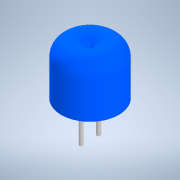
# Autodesk Inventor part: LED
Saved by Autodesk Inventor 2021 (Build 250183000, 183)
## iProperties
Created: 2021-06-29
Part Number: LED
Material: Generic
Document SubType Name: Modeling
Designer: shifa
Density: 1 g/cm^3
Appearance: Default
Author: shifa
Autodesk Inventor part; units mm, degrees
ref_plane "YZ Plane" through (0, 0, 0) normal (1, 0, 0) x (0, 1, 0)
ref_plane "XZ Plane" through (0, 0, 0) normal (0, 1, 0) x (-1, 0, 0)
ref_plane "XY Plane" through (0, 0, 0) normal (0, 0, 1) x (1, 0, 0)
sketch "Sketch1" plane through (0, 0, 0) normal (0, 0, 1) x (1, 0, 0)
  line L0 (3, -6.7347) -> (-5, -6.7347)
  line L1 (-5, -6.7347) -> (-5, 3.2653)
  line L2 (-1, 7.2653) -> (-1, 7.2653)
  line L3 (3, 3.2653) -> (3, -6.7347)
  arc A0 (3, 3.2653) -> (-1, 7.2653) centre (-1, 3.2653) ccw
  arc A1 (-1, 7.2653) -> (-5, 3.2653) centre (-1, 3.2653) ccw
  point P0 (0, 0)
  point P1 (-5, 7.2653)
  point P2 (3, 7.2653)
  point P3 (-1, 7.2653)
  dimension "d0" = 8
  dimension "d1" = 14
  dimension "d2" = 4
  constraints: 8 end point, 4 point on circle, 4 point on line, 4 tangent, 2 centre point, 2 parallel, 1 concentric, 1 horizontal, 1 perpendicular
  measures "d0" distance of point (-5, 7.265) point (3, 7.265)
  measures "d1" distance of L0.end point (-5, 7.265)
  measures "d2" radius of A0
revolve "Revolution1" add sketch "Sketch1" angle 360 about axis through (3, 3.2653, 0) along (0, -1, 0)
sketch "Sketch2" plane through (3, -6.7347, 0) normal (0, -1, 0) x (1, 0, 0)
  circle A0 centre (0, 2.4175) radius 0.5
  circle A1 centre (0, -2.4175) radius 0.5
  point P0 (-3, 0)
  dimension "d4" = 1
  dimension "d5" = 1
  dimension "d8" = 4.8351
  constraints: 2 centre point
  measures "d4" diameter of A0
  measures "d5" diameter of A1
  measures "d8" distance of A1.centre A0.centre
sketch "Sketch3" plane through (3, -6.7347, 0) normal (0, -1, 0) x (1, 0, 0)
  point P0 (-3, 0)
extrude "Extrusion1" add sketch "Sketch2" along normal blind 10
body "Solid1"
